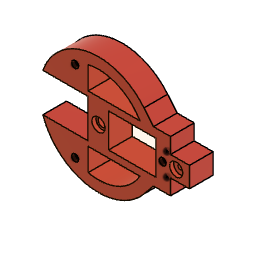
colosseum_baseplate (Autodesk Fusion 360 design; units mm, degrees)
Autodesk Fusion 360 part; units mm, degrees
sketch "Sketch1" plane through (0, 0, 0) normal (0, 1, 0) x (1, 0, 0)
  circle A0 centre (-34.5, 59.7558) radius 3.5
  circle A1 centre (-34.5, -59.7558) radius 3.5
  circle A2 centre (95, 0) radius 3.5
  circle A3 centre (0, 0) radius 9.75
  circle A4 centre (115, 0) radius 9.75
  arc A5 (64.6488, -61.1681) -> (68.8783, -56.363) centre (0, 0) ccw
  line L0 (68.8783, -56.363) -> (82.2681, -40)
  line L1 (82.2681, -40) -> (136.6025, -40)
  line L2 (136.6025, -40) -> (136.6025, 40)
  line L3 (136.6025, 40) -> (82.2681, 40)
  line L4 (82.2681, 40) -> (68.8783, 56.363)
  arc A6 (68.8783, 56.363) -> (64.6488, 61.1681) centre (0, 0) ccw
  arc A7 (20.6487, 86.5715) -> (10.2058, 88.4129) centre (0, 0) ccw
  arc A8 (-39.8293, 79.5904) -> (-49.0127, 74.2884) centre (0, 0) ccw
  arc A9 (-81.6707, 35.368) -> (-85.2975, 25.4035) centre (0, 0) ccw
  arc A10 (-85.2975, -25.4035) -> (-81.6707, -35.368) centre (0, 0) ccw
  arc A11 (-49.0127, -74.2884) -> (-39.8293, -79.5904) centre (0, 0) ccw
  arc A12 (10.2058, -88.4129) -> (20.6487, -86.5715) centre (0, 0) ccw
  arc A13 (68.8783, 56.363) -> (68.8783, -56.363) centre (0, 0) ccw
  line L5 (-15.7, -25) -> (-65.7, -25) construction
  line L6 (-65.7, -25) -> (-65.7, 25) construction
  line L7 (-65.7, 25) -> (-15.7, 25) construction
  line L8 (-15.7, 25) -> (-15.7, -25) construction
  line L9 (-15.7, -25) -> (-65.7, 25) construction
  line L10 (-65.7, -25) -> (-15.7, 25) construction
  line L11 (-15.7, 25) -> (-15.7, -25)
  circle A14 centre (0, 0) radius 6.5
  circle A15 centre (115, 0) radius 3.4
  line L12 (85, -25) -> (15, -25)
  line L13 (15, -25) -> (15, 25)
  line L14 (15, 25) -> (85, 25)
  line L15 (85, 25) -> (85, -25)
  line L16 (85, -25) -> (15, 25) construction
  line L17 (15, -25) -> (85, 25) construction
  line L18 (-15.7, -25) -> (-15.7, -56.7134)
  line L19 (-15.7, 25) -> (-15.7, 56.7134)
  arc A16 (-15.3174, -69.1766) -> (-15.3174, 69.1766) centre (0, 0) ccw
  line L20 (-15.3174, 69.1766) -> (-15.3174, -69.1766)
  line L21 (-15.3174, -35.4897) -> (61.3229, -35.4897)
  line L22 (-15.3174, 35.4897) -> (61.3229, 35.4897)
  circle A17 centre (47.5257, -69.2626) radius 2.75
  circle A18 centre (115, -25) radius 2.75
  circle A19 centre (-84, 0) radius 2.75
  circle A20 centre (47.5257, 69.2626) radius 2.75
  circle A21 centre (115, 25) radius 2.75
  line L23 (136.6025, 40) -> (106.6025, 40)
  line L24 (106.6025, 40) -> (106.6025, 15)
  line L25 (106.6025, 15) -> (136.6025, 15)
  line L26 (136.6025, 15) -> (136.6025, 40)
  line L27 (136.6025, -40) -> (106.6025, -40)
  line L28 (106.6025, -40) -> (106.6025, -15)
  line L29 (106.6025, -15) -> (136.6025, -15)
  line L30 (136.6025, -15) -> (136.6025, -40)
  arc A22 (67.3304, 55.0964) -> (67.3304, -55.0964) centre (0, 0) ccw
  line L31 (67.3304, -55.0964) -> (81.3204, -38)
  line L32 (81.3204, -38) -> (134.6025, -38)
  line L33 (134.6025, -38) -> (134.6025, 38)
  line L34 (134.6025, 38) -> (81.3204, 38)
  line L35 (81.3204, 38) -> (67.3304, 55.0964)
  line L36 (-15.7, 28.5002) -> (-82.1994, 28.5002)
  line L37 (-15.7, -28.4897) -> (-82.203, -28.4897)
  line L38 (-46.7, 12.5) -> (-38.7, 12.5)
  arc A23 (-38.7, -12.5) -> (-38.7, 12.5) centre (-38.7, 0) ccw
  line L39 (-38.7, -12.5) -> (-46.7, -12.5)
  arc A24 (-46.7, 12.5) -> (-46.7, -12.5) centre (-46.7, 0) ccw
  arc A25 (-23.2, -18) -> (-23.2, -13) centre (-23.2, -15.5) ccw
  line L40 (-23.2, -18) -> (-31.2, -18)
  arc A26 (-31.2, -13) -> (-31.2, -18) centre (-31.2, -15.5) ccw
  line L41 (-31.2, -13) -> (-23.2, -13)
  arc A27 (-54.2, 13) -> (-54.2, 18) centre (-54.2, 15.5) ccw
  line L42 (-54.2, 13) -> (-62.2, 13)
  arc A28 (-62.2, 18) -> (-62.2, 13) centre (-62.2, 15.5) ccw
  line L43 (-62.2, 18) -> (-54.2, 18)
  arc A29 (-23.2, 13) -> (-23.2, 18) centre (-23.2, 15.5) ccw
  line L44 (-23.2, 13) -> (-31.2, 13)
  arc A30 (-31.2, 18) -> (-31.2, 13) centre (-31.2, 15.5) ccw
  line L45 (-31.2, 18) -> (-23.2, 18)
  arc A31 (-54.2, -18) -> (-54.2, -13) centre (-54.2, -15.5) ccw
  line L46 (-54.2, -18) -> (-62.2, -18)
  arc A32 (-62.2, -13) -> (-62.2, -18) centre (-62.2, -15.5) ccw
  line L47 (-62.2, -13) -> (-54.2, -13)
  point P0 (-40.7, 0)
  point P1 (50, 0)
  dimension "d1827" = 50
  dimension "d1828" = 50
  dimension "d1829" = 13
  dimension "d1830" = 6.8
  dimension "d1871" = 70
  dimension "d1872" = 50
  dimension "d1875" = 50
  dimension "d1876" = 65
  dimension "d1879" = 33.6868
  dimension "d1880" = 33.6868
  dimension "d1881" = 70.8521
  dimension "d1882" = 138.3531
  dimension "d2112" = 25
  dimension "d2113" = 30
  dimension "d2114" = 30
  dimension "d2115" = 25
  dimension "d2118" = 30
  dimension "d2119" = 25
  dimension "d2120" = 25
  dimension "d2121" = 30
  dimension "d2122" = -2
  dimension "d2175" = 7
  dimension "d2177" = 16.1479
  dimension "d2178" = 7
  constraint perpendicular L5 L6
  constraint parallel L5 L7
  constraint parallel L6 L8
  constraint horizontal L5
  constraint coincident L9 P0
  constraint coincident L10 P0
  constraint concentric A3 A14
  constraint concentric A4 A15
  constraint perpendicular L12 L13
  constraint parallel L12 L14
  constraint parallel L13 L15
  constraint horizontal L12
  constraint coincident L16 P1
  constraint coincident L17 P1
  constraint perpendicular L5 L18
  constraint perpendicular L7 L19
  constraint coincident A3.centre A5.centre
  constraint vertical L20
  constraint coincident L20 L21.start
  constraint coincident A16 L21.end
  constraint perpendicular L20 L21
  constraint coincident L20 L22.start
  constraint coincident A16 L22.end
  constraint perpendicular L20 L22
  constraint horizontal L23
  constraint vertical L24
  constraint horizontal L25
  constraint vertical L26
  constraint horizontal L27
  constraint vertical L28
  constraint horizontal L29
  constraint vertical L30
  constraint coincident L19 L36.start
  constraint coincident A22 L36.end
  constraint perpendicular L19 L36
  constraint coincident L18 L37.start
  constraint coincident A22 L37.end
  constraint perpendicular L18 L37
  measures "d1827" distance of L5.end L6.end
  measures "d1828" distance of L6.end L7.end
  measures "d1829" diameter of A14
  measures "d1830" diameter of A15
  measures "d1871" distance of L13.end L14.end
  measures "d1872" distance of L12.end L13.end
  measures "d1875" distance of A3.centre P1
  measures "d1876" distance of A4.centre P1
  measures "d1879" distance of A16.start L21.start
  measures "d1880" distance of A16.end L22.start
  measures "d1881" distance of A3.centre A16.end
  measures "d1882" distance of A16.end A16.start
  measures "d2112" distance of L23.end L24.end
  measures "d2113" distance of L24.end L25.end
  measures "d2114" distance of L28.end L29.end
  measures "d2115" distance of L27.end L28.end
  measures "d2118" distance of L2 L28
  measures "d2119" distance of L1 L29
  measures "d2120" distance of L3 L25
  measures "d2121" distance of L2 L24
  measures "d2175" vertical distance of L21.start L37.start
  measures "d2177" distance of A16 A22
  measures "d2178" distance of L22.start L36.start
extrude "Extrude1" add sketch "Sketch1" along normal blind 35 contours A0 | A1 | A2 | A3 | A4 | L11 L18 L19 L24 L25 L28 L29 A22 L31 L32 L33 L34 L35 L36 L37 | L12 L13 L14 A16 L20 L21 L22 | A17 | A20
extrude "Extrude2" cut sketch "Sketch1" along normal blind 6 contours A3 | A4
sketch "Sketch3" plane through (0, 35, 0) normal (0, 1, 0) x (-1, 0, 0)
  arc A0 (15.3174, 69.1766) -> (-61.3229, 35.4897) centre (0, 0) ccw
  line L0 (15.3174, 69.1766) -> (15.3174, 35.4897)
  line L1 (15.3174, 35.4897) -> (-61.3229, 35.4897)
  line L2 (-61.3229, -35.4897) -> (15.3174, -35.4897)
  line L3 (15.3174, -35.4897) -> (15.3174, -69.1766)
  arc A1 (-61.3229, -35.4897) -> (15.3174, -69.1766) centre (0, 0) ccw
  line L4 (-15, -25) -> (-85, -25)
  line L5 (-85, -25) -> (-85, 25)
  line L6 (-85, 25) -> (-15, 25)
  line L7 (-15, 25) -> (-15, -25)
  circle A2 centre (0, 0) radius 6.5
  circle A3 centre (-115, 0) radius 3.4
  line L8 (15.7, -28.5002) -> (15.7, 28.4897)
  line L9 (15.7, 28.4897) -> (82.203, 28.4897)
  arc A4 (82.203, 28.4897) -> (-67.3304, 55.0964) centre (0, 0) ccw
  line L10 (-67.3304, 55.0964) -> (-81.3204, 38)
  line L11 (-81.3204, 38) -> (-106.6025, 38)
  line L12 (-106.6025, 38) -> (-106.6025, 15)
  line L13 (-106.6025, 15) -> (-134.6025, 15)
  line L14 (-134.6025, 15) -> (-134.6025, -15)
  line L15 (-134.6025, -15) -> (-106.6025, -15)
  line L16 (-106.6025, -15) -> (-106.6025, -38)
  line L17 (-106.6025, -38) -> (-81.3204, -38)
  line L18 (-81.3204, -38) -> (-67.3304, -55.0964)
  arc A5 (-67.3304, -55.0964) -> (82.1994, -28.5002) centre (0, 0) ccw
  line L19 (82.1994, -28.5002) -> (15.7, -28.5002)
  circle A6 centre (34.5, -59.7558) radius 3.5
  circle A7 centre (34.5, 59.7558) radius 3.5
  circle A8 centre (-95, 0) radius 3.5
extrude "Extrude4" cut sketch "Sketch3" against normal up to surface (35 mm away) contours A6 | A7 | A8
sketch "Sketch4" plane through (0, 0, 0) normal (0, -1, 0) x (1, 0, 0)
  circle A0 centre (-34.5, 59.7558) radius 3.5
  circle A1 centre (95, 0) radius 3.5
  circle A2 centre (-34.5, -59.7558) radius 3.5
  circle A3 centre (115, 0) radius 9.75
  circle A4 centre (0, 0) radius 9.75
  line L0 (-15.3174, -35.4897) -> (61.3229, -35.4897)
  arc A5 (-15.3174, -69.1766) -> (61.3229, -35.4897) centre (0, 0) ccw
  line L1 (-15.3174, -69.1766) -> (-15.3174, -35.4897)
  line L2 (85, -25) -> (15, -25)
  line L3 (15, -25) -> (15, 25)
  line L4 (15, 25) -> (85, 25)
  line L5 (85, 25) -> (85, -25)
  arc A6 (61.3229, 35.4897) -> (-15.3174, 69.1766) centre (0, 0) ccw
  line L6 (61.3229, 35.4897) -> (-15.3174, 35.4897)
  line L7 (-15.3174, 35.4897) -> (-15.3174, 69.1766)
  line L8 (-15.7, 28.4897) -> (-15.7, -28.5002)
  line L9 (-15.7, -28.5002) -> (-82.1994, -28.5002)
  arc A7 (-82.1994, -28.5002) -> (67.3304, -55.0964) centre (0, 0) ccw
  line L10 (67.3304, -55.0964) -> (81.3204, -38)
  line L11 (81.3204, -38) -> (106.6025, -38)
  line L12 (106.6025, -38) -> (106.6025, -15)
  line L13 (106.6025, -15) -> (134.6025, -15)
  line L14 (134.6025, -15) -> (134.6025, 15)
  line L15 (134.6025, 15) -> (106.6025, 15)
  line L16 (106.6025, 15) -> (106.6025, 38)
  line L17 (106.6025, 38) -> (81.3204, 38)
  line L18 (81.3204, 38) -> (67.3304, 55.0964)
  arc A8 (67.3304, 55.0964) -> (-82.203, 28.4897) centre (0, 0) ccw
  line L19 (-82.203, 28.4897) -> (-15.7, 28.4897)
  circle A9 centre (-34.5, 59.7558) radius 5
  circle A10 centre (-34.5, -59.7558) radius 5
  circle A11 centre (95, 0) radius 5
  circle A12 centre (101.6025, 16.5) radius 1
  circle A13 centre (101.6025, -16.5) radius 1
  dimension "d2298" = 10
  dimension "d2299" = 10
  dimension "d2300" = 10
  dimension "d2303" = 2
  dimension "d2304" = 5
  dimension "d2305" = 21.5
  dimension "d2308" = 2
  dimension "d2309" = 5
  dimension "d2310" = 21.5
  constraint concentric A0 A9
  constraint concentric A2 A10
  constraint concentric A1 A11
  measures "d2298" diameter of A9
  measures "d2299" diameter of A10
  measures "d2300" diameter of A11
  measures "d2303" diameter of A12
  measures "d2304" distance of L16 A12.centre
  measures "d2305" distance of L17 A12.centre
  measures "d2308" diameter of A13
  measures "d2309" distance of L12 A13.centre
  measures "d2310" distance of L11 A13.centre
extrude "Extrude5" cut sketch "Sketch4" against normal blind 5 contours A9 | A10 | A11
extrude "Extrude6" cut sketch "Sketch4" against normal up to surface (35 mm away) contours A12 | A13
